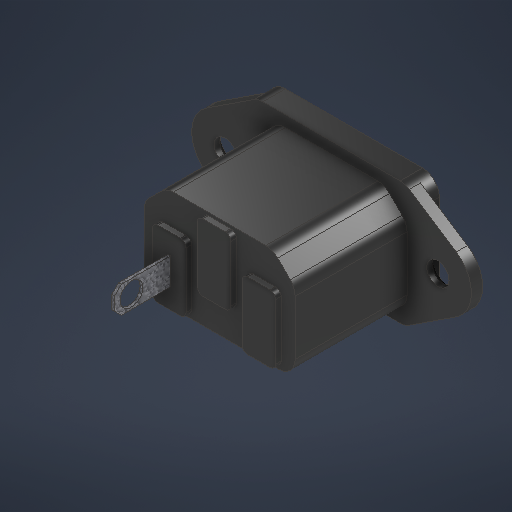
# Autodesk Inventor part: my_C14
Saved by Autodesk Inventor 2026 (Build 300175000, 175)
## iProperties
Created: 2025-05-21
Part Number: my_C14
Material: Generic
Document SubType Name: Modeling
Designer: Paul Juschitz
Density: 1 g/cm^3
Appearance: Knurled 45
c14_inside_outer_width: 27,000 mm
c14_inside_outer_height: 18,000 mm
c14_inner_depth: 20,000 mm
c14_inner_chamfer: 4,000 mm
c14_outer_width_1: 30,500 mm
c14_outer_height: 22,000 mm
c14_outer_fillet: 3,000 mm
c14_inner_fillet: 0,500 mm
Author: Paul Juschitz
Autodesk Inventor part; units mm, degrees
ref_plane "YZ Plane" through (0, 0, 0) normal (1, 0, 0) x (0, 1, 0)
ref_plane "XZ Plane" through (0, 0, 0) normal (0, 1, 0) x (-1, 0, 0)
ref_plane "XY Plane" through (0, 0, 0) normal (0, 0, 1) x (1, 0, 0)
sketch "Sketch1" plane through (0, 0, 0) normal (0, 0, 1) x (1, 0, 0)
  line L0 (-13.5, 9) -> (13.5, 9)
  line L1 (13.5, 9) -> (13.5, -9)
  line L2 (13.5, -9) -> (-13.5, -9)
  line L3 (-13.5, -9) -> (-13.5, 9)
  line L4 (-13.5, 9) -> (13.5, -9) construction
  line L5 (13.5, 9) -> (-13.5, -9) construction
  point P0 (0, 0)
  dimension "c14_inside_outer_width" = 27
  dimension "c14_inside_outer_height" = 18
  constraints: 12 end point, 2 midpoint, 2 parallel, 1 horizontal, 1 perpendicular
  measures "c14_inside_outer_width" distance of L1.end L2.end
  measures "c14_inside_outer_height" distance of L0.end L1.end
extrude "Extrusion1" add sketch "Sketch1" along normal blind 20
chamfer "Chamfer1" distance 4 angle 45 2 edges at (-13.5, 9, 10) (13.5, 9, 10)
sketch "Sketch2" plane through (0, 0, 20) normal (0, 0, 1) x (1, 0, 0)
  line L0 (-2, 8.5) -> (2, 8.5)
  line L1 (3, 7.5) -> (3, -2.5)
  line L2 (2, -3.5) -> (-2, -3.5)
  line L3 (-3, -2.5) -> (-3, 7.5)
  line L4 (-3, 8.5) -> (3, -3.5) construction
  line L5 (3, 8.5) -> (-3, -3.5) construction
  line L6 (9.5, 9) -> (-9.5, 9) construction
  line L7 (0, 9) -> (0, -9)
  line L8 (-13.5, -9) -> (13.5, -9) construction
  arc A0 (-2, 8.5) -> (-3, 7.5) centre (-2, 7.5) ccw
  arc A1 (3, 7.5) -> (2, 8.5) centre (2, 7.5) ccw
  arc A2 (2, -3.5) -> (3, -2.5) centre (2, -2.5) ccw
  arc A3 (-3, -2.5) -> (-2, -3.5) centre (-2, -2.5) ccw
  line L9 (-10, 3.5) -> (-6, 3.5)
  line L10 (-5, 2.5) -> (-5, -7.5)
  line L11 (-6, -8.5) -> (-10, -8.5)
  line L12 (-11, -7.5) -> (-11, 2.5)
  line L13 (-11, 3.5) -> (-5, -8.5) construction
  line L14 (-5, 3.5) -> (-11, -8.5) construction
  arc A4 (-10, 3.5) -> (-11, 2.5) centre (-10, 2.5) ccw
  arc A5 (-5, 2.5) -> (-6, 3.5) centre (-6, 2.5) ccw
  arc A6 (-6, -8.5) -> (-5, -7.5) centre (-6, -7.5) ccw
  arc A7 (-11, -7.5) -> (-10, -8.5) centre (-10, -7.5) ccw
  line L15 (6, -8.5) -> (10, -8.5)
  arc A8 (10, -8.5) -> (11, -7.5) centre (10, -7.5) ccw
  line L16 (5, 2.5) -> (5, -7.5)
  line L17 (11, -7.5) -> (11, 2.5)
  line L18 (11, 3.5) -> (5, -8.5) construction
  line L19 (5, 3.5) -> (11, -8.5) construction
  arc A9 (6, 3.5) -> (5, 2.5) centre (6, 2.5) ccw
  line L20 (10, 3.5) -> (6, 3.5)
  arc A10 (11, 2.5) -> (10, 3.5) centre (10, 2.5) ccw
  arc A11 (5, -7.5) -> (6, -8.5) centre (6, -7.5) ccw
  point P0 (0, 0)
  point P1 (0, 2.5)
  point P2 (-8, -2.5)
  point P3 (8, -2.5)
  dimension "d7" = 6
  dimension "d8" = 12
  dimension "d9" = 0.5
  dimension "d10" = 1
  dimension "d11" = 6
  dimension "d12" = 12
  dimension "d13" = 1
  dimension "d14" = 0.5
  dimension "d15" = 2
  constraints: 38 end point, 25 point on line, 24 point on circle, 17 symmetric about line, 16 tangent, 12 centre point, 6 equal radius, 6 midpoint, 4 parallel, 2 horizontal, 2 perpendicular, 4 other
  measures "d7" distance of L4.end L5.end
  measures "d8" distance of L5.start L4.end
  measures "d9" distance between parallel lines of L6 L0
  measures "d10" radius of A0
  measures "d11" distance of L13.end L14.end
  measures "d12" distance of L14.start L13.end
  measures "d13" radius of A4
  measures "d14" distance between parallel lines of L8 L11
  measures "d15" distance between parallel lines of L3 L10
extrude "Extrusion2" add sketch "Sketch2" along normal blind 1
sketch "Sketch3" plane through (0, 0, 0) normal (0, 0, -1) x (-1, 0, 0)
  line L0 (-13.5, 5) -> (-9.5, 9) construction
  line L1 (-13.5, -9) -> (-13.5, 5) construction
  line L2 (13.5, -9) -> (-13.5, -9) construction
  line L3 (13.5, 5) -> (13.5, -9) construction
  line L4 (9.5, 9) -> (13.5, 5) construction
  line L5 (-9.5, 9) -> (9.5, 9) construction
  line L6 (0, 9) -> (0, -9)
  line L7 (-15.25, 11) -> (15.25, 11)
  line L8 (15.25, 11) -> (15.25, -11)
  line L9 (15.25, -11) -> (-15.25, -11)
  line L10 (-15.25, -11) -> (-15.25, 11)
  line L11 (-15.25, 11) -> (15.25, -11) construction
  line L12 (15.25, 11) -> (-15.25, -11) construction
  line L13 (-13.5, -9) -> (-13.5, 9) construction
  line L14 (-13.5, 0) -> (13.5, 0) construction
  point P0 (0, 0)
  point P1 (0, 0)
  dimension "c14_outer_width_1" = 30.5
  dimension "c14_outer_height" = 22
  constraints: 18 end point, 7 midpoint, 2 parallel, 2 perpendicular, 1 horizontal, 1 horizontal alignment, 1 point on line, 1 vertical
  measures "c14_outer_width_1" distance of L8.end L9.end
  measures "c14_outer_height" distance of L7.end L8.end
extrude "Extrusion3" add sketch "Sketch3" along normal blind 4
fillet "Fillet1" radius 3 4 edges at (-15.25, 11, -2) (-15.25, -11, -2) (15.25, -11, -2) (15.25, 11, -2)
sketch "Sketch5" plane through (0, 0, 0) normal (0, 0, 1) x (1, 0, 0)
  line L0 (-12.25, 11) -> (12.25, 11) projected
  arc A0 (-12.25, 11) -> (-15.25, 8) centre (-12.25, 8) ccw construction
  line L1 (-15.25, -8) -> (-15.25, 8) construction
  arc A1 (-15.25, -8) -> (-12.25, -11) centre (-12.25, -8) ccw construction
  line L2 (12.25, -11) -> (-12.25, -11) projected
  arc A2 (12.25, -11) -> (15.25, -8) centre (12.25, -8) ccw construction
  line L3 (15.25, 8) -> (15.25, -8) construction
  arc A3 (15.25, 8) -> (12.25, 11) centre (12.25, 8) ccw construction
  line L4 (0, 11) -> (0, -11)
  arc A4 (-12.25, 11) -> (-13.8922, 10.5106) centre (-12.25, 8) ccw
  line L5 (-13.8922, 10.5106) -> (-22.2844, 5.0212)
  line L6 (-15.25, 0) -> (15.25, 0)
  arc A5 (-22.2844, 5.0212) -> (-25, 0) centre (-19, 0) ccw
  line L7 (-15.25, 0) -> (-70.2247, 0)
  arc A6 (-13.8922, -10.5106) -> (-12.25, -11) centre (-12.25, -8) ccw
  line L8 (-13.8922, -10.5106) -> (-22.2844, -5.0212)
  arc A7 (-25, 0) -> (-22.2844, -5.0212) centre (-19, 0) ccw
  arc A8 (13.8922, 10.5106) -> (12.25, 11) centre (12.25, 8) ccw
  line L9 (13.8922, 10.5106) -> (22.2844, 5.0212)
  arc A9 (25, 0) -> (22.2844, 5.0212) centre (19, 0) ccw
  arc A10 (12.25, -11) -> (13.8922, -10.5106) centre (12.25, -8) ccw
  line L10 (13.8922, -10.5106) -> (22.2844, -5.0212)
  arc A11 (22.2844, -5.0212) -> (25, 0) centre (19, 0) ccw
  point P0 (0, 0)
  dimension "d26" = 50
  dimension "d27" = 3
  dimension "d28" = 6
  constraints: 16 point on circle, 14 end point, 11 symmetric about line, 8 centre point, 4 midpoint, 3 tangent, 2 point on line, 1 horizontal, 6 other
  measures "d26" distance of A9.start A5.end
  measures "d27" radius of A4
  measures "d28" radius of A7
extrude "Extrusion5" add sketch "Sketch5" against normal blind 2
sketch "Sketch6" plane through (0, 0, -2) normal (0, 0, -1) x (-1, 0, 0)
  arc A0 (22.2844, -5.0212) -> (22.2844, 5.0212) centre (19, 0) ccw construction
  arc A1 (-22.2844, 5.0212) -> (-22.2844, -5.0212) centre (-19, 0) ccw construction
  point P0 (0, 0)
hole "Hole1" at (19, 0, -2) at (-19, 0, -2) direction (0, 0, 1) diameter 4 end through all countersink diameter 6 countersink angle 90
fillet "Fillet3" radius 3 6 edges at (-13.5, 5, 10) (-9.5, 9, 10) (-13.5, -9, 10) (13.5, -9, 10) (13.5, 5, 10) (9.5, 9, 10)
sketch "Sketch7" plane through (0, 0, -4) normal (0, 0, -1) x (-1, 0, 0)
  line L0 (10.5, -9) -> (-10.5, -9) construction
  arc A0 (-13.5, -6) -> (-10.5, -9) centre (-10.5, -6) ccw construction
  line L1 (-13.5, -6) -> (-13.5, 3.7574) construction
  arc A1 (-12.6213, 5.8787) -> (-13.5, 3.7574) centre (-10.5, 3.7574) ccw construction
  line L2 (-10.3787, 8.1213) -> (-12.6213, 5.8787) construction
  arc A2 (-8.2574, 9) -> (-10.3787, 8.1213) centre (-8.2574, 6) ccw construction
  line L3 (-8.2574, 9) -> (8.2574, 9) construction
  arc A3 (10.3787, 8.1213) -> (8.2574, 9) centre (8.2574, 6) ccw construction
  line L4 (12.6213, 5.8787) -> (10.3787, 8.1213) construction
  arc A4 (13.5, 3.7574) -> (12.6213, 5.8787) centre (10.5, 3.7574) ccw construction
  line L5 (13.5, 3.7574) -> (13.5, -6) construction
  arc A5 (10.5, -9) -> (13.5, -6) centre (10.5, -6) ccw construction
  arc A6 (-11.9142, 5.1716) -> (-12.5, 3.7574) centre (-10.5, 3.7574) ccw
  line L6 (-12.5, 3.7574) -> (-12.5, -6)
  arc A7 (-12.5, -6) -> (-10.5, -8) centre (-10.5, -6) ccw
  line L7 (-10.5, -8) -> (10.5, -8)
  arc A8 (10.5, -8) -> (12.5, -6) centre (10.5, -6) ccw
  line L8 (12.5, -6) -> (12.5, 3.7574)
  arc A9 (12.5, 3.7574) -> (11.9142, 5.1716) centre (10.5, 3.7574) ccw
  line L9 (11.9142, 5.1716) -> (9.6716, 7.4142)
  arc A10 (9.6716, 7.4142) -> (8.2574, 8) centre (8.2574, 6) ccw
  line L10 (8.2574, 8) -> (-8.2574, 8)
  arc A11 (-8.2574, 8) -> (-9.6716, 7.4142) centre (-8.2574, 6) ccw
  line L11 (-9.6716, 7.4142) -> (-11.9142, 5.1716)
  point P0 (0, 0)
  dimension "d40" = 1
  constraints: 12 end point, 12 point on circle, 6 centre point, 11 other
  measures "d40" distance between parallel lines of L2 L11
extrude "Extrusion6" cut sketch "Sketch7" against normal blind 21
fillet "Fillet4" radius 0.5 12 edges at (0, 8, -4) (-9.0227, 7.8478, -4) (-10.7929, 6.2929, -4) (-12.3478, 4.5227, -4) (-12.5, -1.1213, -4) (-11.9142, -7.4142, -4) (0, -8, -4) (11.9142, -7.4142, -4) (12.5, -1.1213, -4) (12.3478, 4.5227, -4) (10.7929, 6.2929, -4) (9.0227, 7.8478, -4)
sketch "Sketch8" plane through (0, 0, 21) normal (0, 0, 1) x (1, 0, 0)
  line L0 (-6, 3.5) -> (-10, 3.5) construction
  arc A0 (-10, 3.5) -> (-11, 2.5) centre (-10, 2.5) ccw construction
  line L1 (-11, 2.5) -> (-11, -7.5) construction
  arc A1 (-11, -7.5) -> (-10, -8.5) centre (-10, -7.5) ccw construction
  line L2 (-10, -8.5) -> (-6, -8.5) construction
  arc A2 (-6, -8.5) -> (-5, -7.5) centre (-6, -7.5) ccw construction
  line L3 (-5, -7.5) -> (-5, 2.5) construction
  arc A3 (-5, 2.5) -> (-6, 3.5) centre (-6, 2.5) ccw construction
  line L4 (-8, 3.5) -> (-8, -8.5)
  line L5 (-11, -2.5) -> (-5, -2.5)
  line L6 (-8.25, -0.1) -> (-7.75, -0.1)
  line L7 (-7.75, -0.1) -> (-7.75, -4.9)
  line L8 (-7.75, -4.9) -> (-8.25, -4.9)
  line L9 (-8.25, -4.9) -> (-8.25, -0.1)
  line L10 (-8.25, -0.1) -> (-7.75, -4.9) construction
  line L11 (-7.75, -0.1) -> (-8.25, -4.9) construction
  point P0 (0, 0)
  point P1 (-8, -2.5)
  dimension "d44" = 0.5
  dimension "d45" = 4.8
  constraints: 16 end point, 7 midpoint, 2 parallel, 1 horizontal, 1 perpendicular
  measures "d44" distance of L7.end L8.end
  measures "d45" distance of L6.end L7.end
extrude "Extrusion7" add sketch "Sketch8" along normal blind 10
chamfer "Chamfer2" distance 1.2 angle 45 2 edges at (-8, -0.1, 31) (-8, -4.9, 31)
sketch "Sketch9" plane through (-7.75, -4.9, 21) normal (1, 0, 0) x (0, 0, -1)
  line L0 (-10, 1.2) -> (-10, 3.6) construction
  line L1 (-10, 2.4) -> (0.0273, 2.4)
  circle A0 centre (-7, 2.4) radius 2.05
  point P0 (21, 4.9)
  dimension "d51" = 4.1
  dimension "d52" = 3
  constraints: 2 end point, 1 centre point, 1 horizontal, 1 midpoint, 1 point on line
  measures "d51" diameter of A0
  measures "d52" distance from line of L0 A0.centre
extrude "Extrusion8" cut sketch "Sketch9" against normal blind 10
equation "\"d27\" = c14_outer_fillet"
equation "\"d39\" = c14_outer_fillet"
equation "\"c14_outer_fillet\" = 3"
body "Solid1"
